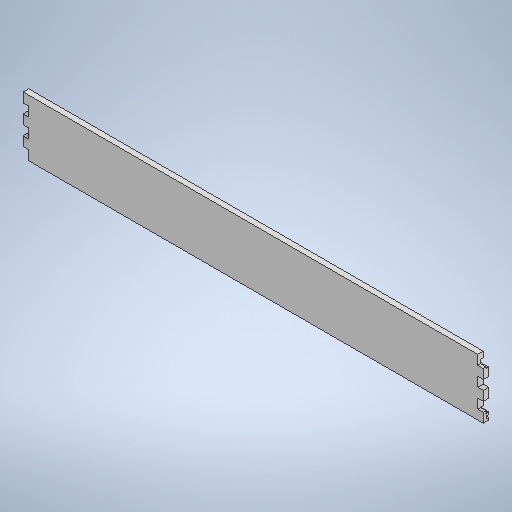
# Autodesk Inventor part: Side Wall
Saved by Autodesk Inventor 2025.2 (Build 292293000, 293)
## iProperties
Created: 2025-04-21
Part Number: Side Wall
Material: Generic
Document SubType Name: Modeling
Designer: powel
Density: 1 g/cm^3
Appearance: Default
Author: powel
Autodesk Inventor part; units mm, degrees
ref_plane "YZ Plane" through (0, 0, 0) normal (1, 0, 0) x (0, 1, 0)
ref_plane "XZ Plane" through (0, 0, 0) normal (0, 1, 0) x (-1, 0, 0)
ref_plane "XY Plane" through (0, 0, 0) normal (0, 0, 1) x (1, 0, 0)
sketch "Sketch1" plane through (0, 0, 0) normal (0, 0, 1) x (1, 0, 0)
  line L0 (3.5, 0) -> (288, 0)
  line L1 (288, 36) -> (0, 36)
  line L2 (288, 0) -> (291.5, 0)
  line L3 (291.5, 0) -> (291.5, 6)
  line L4 (291.5, 6) -> (288, 6)
  line L5 (288, 6) -> (288, 12)
  line L6 (288, 12) -> (291.5, 12)
  line L7 (291.5, 12) -> (291.5, 18)
  line L8 (291.5, 18) -> (288, 18)
  line L9 (288, 18) -> (288, 24)
  line L10 (288, 30) -> (288, 36)
  line L11 (288, 24) -> (291.5, 24)
  line L12 (291.5, 24) -> (291.5, 30)
  line L13 (291.5, 30) -> (288, 30)
  line L14 (0, 36) -> (0, 30)
  line L15 (0, 24) -> (0, 18)
  line L16 (0, 12) -> (0, 6)
  line L17 (0, 30) -> (3.5, 30)
  line L18 (3.5, 30) -> (3.5, 24)
  line L19 (3.5, 24) -> (0, 24)
  line L20 (0, 18) -> (3.5, 18)
  line L21 (3.5, 18) -> (3.5, 12)
  line L22 (3.5, 12) -> (0, 12)
  line L23 (0, 6) -> (3.5, 6)
  line L24 (3.5, 6) -> (3.5, 0)
  line L25 (3.5, 0) -> (291.5, 0)
  line L26 (291.5, 0) -> (291.5, 1.5)
  line L27 (291.5, 1.5) -> (3.5, 1.5)
  line L28 (3.5, 1.5) -> (3.5, 0)
  line L29 (291.5, 1.5) -> (3.5, 1.5)
  line L30 (3.5, 1.5) -> (3.5, 3)
  line L31 (3.5, 3) -> (291.5, 3)
  line L32 (291.5, 3) -> (291.5, 1.5)
  line L33 (3.5, 3) -> (291.5, 3)
  line L34 (291.5, 3) -> (291.5, 4.5)
  line L35 (291.5, 4.5) -> (3.5, 4.5)
  line L36 (3.5, 4.5) -> (3.5, 3)
  line L37 (291.5, 4.5) -> (3.5, 4.5)
  line L38 (0, 6) -> (291.5, 6)
  line L39 (291.5, 6) -> (291.5, 4.5)
  line L40 (0, 36) -> (288, 36)
  line L41 (288, 32.5) -> (0, 32.5)
  line L42 (0, 32.5) -> (0, 36)
  line L43 (288, 32.5) -> (0, 32.5)
  line L44 (0, 32.5) -> (0, 30)
  line L45 (3.5, 29) -> (291.5, 29)
  line L46 (291.5, 29) -> (291.5, 30)
  point P0 (3.5, 1.5)
  dimension "d41" = 288
  dimension "d42" = 36
  dimension "d43" = 3.5
  dimension "d44" = 6
  dimension "d45" = 6
  dimension "d46" = 6
  dimension "d47" = 6
  dimension "d48" = 6
  dimension "d49" = 6
  dimension "d56" = 3.5
  dimension "d57" = 1.5
  dimension "d58" = 1.5
  dimension "d59" = 1.5
  constraints: 94 end point, 16 parallel, 13 horizontal, 10 perpendicular, 6 point on line, 1 midpoint
  measures "d41" distance of L1.start L1.end
  measures "d42" distance of L1.start L0.end
  measures "d43" distance of L4.end L3.end
  measures "d44" distance of L3.end L2.end
  measures "d45" distance of L4.end L5.end
  measures "d46" distance of L7.end L6.end
  measures "d47" distance of L8.end L9.end
  measures "d48" distance of L9.end L10.start
  measures "d49" distance of L1.start L10.start
  measures "d56" distance of L18.end L19.end
  measures "d57" distance of L26.end L25.end
  measures "d58" distance of L29.end L30.end
  measures "d59" distance of L34.end L33.end
extrude "Extrusion1" add sketch "Sketch1" along normal blind 1.75
extrude "Extrusion2" add sketch "Sketch1" against normal blind 1.75 contours L24 L27 L3 L2 L0 | L24 L35 L3 L31 | L23 L16 L22 L21 L20 L15 L19 L18 L45 L12 L11 L9 L8 L7 L6 L5 L38 | L14 L1 L10 L41
body "Solid1"
